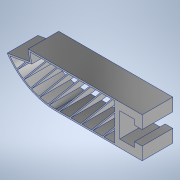
# Autodesk Inventor part: Finray_9_Kerbe_10deg_40deg10inf_PLA
Saved by Autodesk Inventor 2022 (Build 260153000, 153)
## iProperties
Created: 2022-02-28
Part Number: Finray_9_Kerbe_10deg_40deg10inf_PLA
Material: Generic
Document SubType Name: Modeling
Designer: richa
Density: 1 g/cm^3
Appearance: Aluminum - Flat
Author: richa
Autodesk Inventor part; units mm, degrees
ref_plane "YZ Plane" through (0, 0, 0) normal (1, 0, 0) x (0, 1, 0)
ref_plane "XZ Plane" through (0, 0, 0) normal (0, 1, 0) x (-1, 0, 0)
ref_plane "XY Plane" through (0, 0, 0) normal (0, 0, 1) x (1, 0, 0)
sketch "Sketch5" plane through (0, 0, 0) normal (0, 0, 1) x (1, 0, 0)
  line L0 (52.8, -15.6) -> (52.8, -10.6)
  line L1 (52.8, -10.6) -> (49.8, -10.6)
  line L2 (49.8, -10.6) -> (49.8, -12.6)
  line L3 (44, -12.6) -> (44, -3)
  line L4 (49.8, -3) -> (49.8, -5)
  line L5 (49.8, -5) -> (52.8, -5)
  line L6 (52.8, -5) -> (52.8, 0)
  line L7 (52.8, 0) -> (7.8, 0)
  line L8 (44, -3) -> (49.8, -3)
  line L9 (44, -12.6) -> (49.8, -12.6)
  line L10 (52.8, -15.6) -> (7.8, -15.6)
  line L11 (7.8, -15.6) -> (0, -15.6)
  line L12 (0, -15.6) -> (0, 0)
  line L13 (0, 0) -> (7.8, 0)
  point P0 (7.8, 0)
  dimension "d41" = 5.8
  dimension "d48" = 44
  dimension "d50" = 3
  dimension "d63" = 45
  dimension "d71" = 0
  dimension "d87" = 5.6
  dimension "d88" = 9.6
  dimension "d97" = 15.6
  constraints: 28 end point, 8 perpendicular, 4 collinear, 3 parallel, 2 horizontal, 1 vertical
  measures "d41" distance between parallel lines of L2 L3
  measures "d48" distance from line of L3 L12.end
  measures "d50" distance of L4.end L5.end
  measures "d63" distance of L0.start L10.end
  measures "d71" distance from line of L12.end L7
  measures "d87" distance from line of L0.end L5
  measures "d88" distance of L3.start L3.end
  measures "d97" distance of L11.end L12.end
extrude "Extrusion2" add sketch "Sketch5" along normal blind 12
sketch "Sketch8" plane through (0, 0, 0) normal (0, 0, -1) x (-1, 0, 0)
  line L0 (-8.1687, 0) -> (-8.8633, -3.9392)
  line L1 (-7.8, 0) -> (-1.143, 0) construction
  line L2 (0, -5.5021) -> (-8.8633, -3.9392)
  line L3 (-7.8, 0) -> (-8.1687, 0)
  line L4 (0, 0) -> (0, -15.6) projected
  line L5 (-52.8, 0) -> (0, 0) projected
  line L6 (-7.8, 0) -> (0, 0)
  line L7 (0, 0) -> (0, -5.5021)
  dimension "d80" = 100
  dimension "d95" = 4
  dimension "d96" = 9
  constraints: 12 end point, 2 collinear, 2 perpendicular, 1 horizontal, 1 point on line
  measures "d80" angle of L0 L1
  measures "d95" distance of L0.start L0.end
  measures "d96" distance of L2.start L0.end
extrude "Extrusion5" cut sketch "Sketch8" against normal through all
fillet "Fillet2" radius 23 1 edges at (0, -15.6, 6)
shell "Shell1" thickness 0.62 removed faces 1 at (23.9679, -7.5131, 12)
sketch "Sketch13" plane through (0, 0, 12) normal (0, 0, 1) x (1, 0, 0)
  line L0 (19.0404, -15.6) -> (52.8, -15.6) projected
  line L1 (42.0526, -15.6) -> (42.0526, 0)
  line L2 (52.8, 0) -> (8.1687, 0) projected
  line L3 (52.8, 0) -> (8.1687, 0) projected
  line L4 (52.8, -5) -> (52.8, 0) projected
  line L5 (49.8, -5) -> (52.8, -5) projected
  line L6 (49.8, -3) -> (49.8, -5) projected
  line L7 (44, -3) -> (49.8, -3) projected
  line L8 (44, -12.6) -> (44, -3) projected
  line L9 (49.8, -12.6) -> (44, -12.6) projected
  line L10 (49.8, -10.6) -> (49.8, -12.6) projected
  line L11 (52.8, -10.6) -> (49.8, -10.6) projected
  line L12 (52.8, -15.6) -> (52.8, -10.6) projected
  line L13 (42.0526, 0) -> (52.8, 0)
  line L14 (52.8, -5) -> (52.8, 0) projected
  line L15 (52.8, -5) -> (52.8, 0)
  line L16 (52.8, 0) -> (52.8, -5)
  line L17 (44, -12.6) -> (44, -3) projected
  line L18 (44, -3) -> (44, -12.6)
  line L19 (49.8, -12.6) -> (44, -12.6) projected
  line L20 (44, -12.6) -> (49.8, -12.6)
  line L21 (43.38, -13.22) -> (50.42, -13.22) projected
  line L22 (52.8, -10.6) -> (52.8, -15.6)
  line L23 (52.8, -15.6) -> (42.0526, -15.6)
  line L24 (44, -3) -> (49.8, -3) projected
  line L25 (44, -3) -> (49.8, -3)
  line L26 (49.8, -3) -> (49.8, -5)
  line L27 (49.8, -5) -> (52.8, -5)
  line L28 (52.8, -10.6) -> (49.8, -10.6)
  line L29 (49.8, -10.6) -> (49.8, -12.6)
  point P0 (0, 0)
  dimension "d102" = 10.7474
  constraints: 26 end point, 10 collinear, 2 point on line, 2 vertical, 1 parallel
  measures "d102" distance between parallel lines of L4 L1
extrude "Extrusion7" add sketch "Sketch13" against normal blind 12
sketch "Sketch14" plane through (8.9076, -0.62, 0.62) normal (0, 0, 1) x (1, 0, 0)
  line L0 (33.145, -14.36) -> (33.145, 0) projected
  line L1 (33.145, 0) -> (0, 0) projected
  line L2 (0.6739, -3.8221) -> (0, 0) projected
  line L3 (-7.835, -5.3225) -> (0.6739, -3.8221) projected
  arc A0 (-7.835, -5.3225) -> (10.1328, -14.36) centre (10.1328, 8.02) ccw projected
  line L4 (10.1328, -14.36) -> (33.145, -14.36) projected
  point P0 (-8.9076, 0.62)
extrude "Extrusion8" cut sketch "Sketch14" against normal blind 12
sketch "Sketch15" plane through (0, 0, 12) normal (0, 0, 1) x (1, 0, 0)
  line L0 (42.0526, -0.62) -> (8.9076, -0.62) construction
  line L1 (19.0404, -14.98) -> (42.0526, -14.98) projected
  line L2 (49.5848, -0.3757) -> (49.8759, -0.62)
  line L3 (49.8759, -0.62) -> (37.6215, -15.2243)
  line L4 (37.6215, -15.2243) -> (37.3304, -14.98)
  line L5 (37.3304, -14.98) -> (49.5848, -0.3757)
  arc A0 (1.0726, -5.9425) -> (19.0404, -14.98) centre (19.0404, 7.4) ccw projected
  line L6 (42.0526, -0.62) -> (42.0526, -14.98) projected
  line L7 (1.0726, -5.9425) -> (9.5815, -4.4421) projected
  arc A1 (0, -5.5021) -> (19.0404, -15.6) centre (19.0404, 7.4) ccw projected
  line L8 (42.0526, -14.98) -> (19.0404, -14.98) projected
  line L9 (8.9076, -0.62) -> (42.0526, -0.62) projected
  line L10 (45.5759, -0.62) -> (33.5265, -14.98)
  line L11 (45.0799, -0.62) -> (33.0304, -14.98)
  line L12 (36.9759, -0.62) -> (24.9265, -14.98)
  line L13 (36.4799, -0.62) -> (24.4304, -14.98)
  line L14 (32.6759, -0.62) -> (20.6265, -14.98)
  line L15 (32.1799, -0.62) -> (20.1304, -14.98)
  line L16 (28.3759, -0.62) -> (16.3265, -14.98)
  line L17 (27.8799, -0.62) -> (15.8304, -14.98)
  line L18 (24.0759, -0.62) -> (12.7769, -14.0856)
  line L19 (19.7759, -0.62) -> (9.5131, -12.8508)
  line L20 (19.2799, -0.62) -> (9.1597, -12.6807)
  line L21 (15.4759, -0.62) -> (6.5968, -11.2017)
  line L22 (14.9799, -0.62) -> (6.2812, -10.9866)
  line L23 (11.1759, -0.62) -> (3.9997, -9.1723)
  line L24 (10.6799, -0.62) -> (3.7202, -8.9143)
  line L25 (23.5799, -0.62) -> (12.381, -13.9663)
  line L26 (41.2759, -0.62) -> (29.2265, -14.98)
  line L27 (40.7799, -0.62) -> (28.7304, -14.98)
  point P0 (0, 0)
  point P1 (37.3304, -14.98)
  point P2 (7.6887, -4.7759)
  point P3 (7.1065, -4.8786)
  point P4 (37.8265, -14.98)
  point P5 (37.3304, -14.98)
  point P6 (33.0304, -14.98)
  point P7 (33.5265, -14.98)
  point P8 (28.7304, -14.98)
  point P9 (29.2265, -14.98)
  point P10 (24.4304, -14.98)
  point P11 (20.1304, -14.98)
  point P12 (20.6265, -14.98)
  point P13 (19.1926, -14.98)
  point P14 (19.4987, -14.98)
  point P15 (42.0526, -4.8189)
  point P16 (42.0526, -4.2278)
  point P17 (16.004, -14.7731)
  point P18 (16.4524, -14.8299)
  dimension "d105" = 0.38
  dimension "d130" = 130
  dimension "d132" = 130
  dimension "d133" = 0.38
  dimension "d135" = 0.38
  dimension "d136" = 0.38
  dimension "d137" = 0.38
  dimension "d138" = 0.38
  dimension "d139" = 0.38
  dimension "d140" = 0.38
  dimension "d141" = 0.38
  dimension "d143" = 0.38
  dimension "d152" = 130
  dimension "d155" = 4.3
  dimension "d156" = 4.3
  dimension "d157" = 4.3
  dimension "d158" = 4.3
  dimension "d159" = 4.3
  dimension "d160" = 4.3
  dimension "d161" = 4.3
  dimension "d162" = 4.3
  dimension "d164" = 4.3
  constraints: 44 end point, 18 parallel, 4 point on line, 1 perpendicular, 41 other
  measures "d105" distance between parallel lines of L3 L5
  measures "d130" angle of L0 L3
  measures "d132" angle of L0 L10
  measures "d133" distance between parallel lines of L10 L11
  measures "d135" distance between parallel lines of L13 L12
  measures "d136" distance between parallel lines of L15 L14
  measures "d137" distance between parallel lines of L17 L16
  measures "d138" distance between parallel lines of L25 L18
  measures "d139" distance between parallel lines of L20 L19
  measures "d140" distance between parallel lines of L22 L21
  measures "d141" distance between parallel lines of L24 L23
  measures "d143" distance between parallel lines of L26 L27
  measures "d152" angle of L0 L12
  measures "d155" distance of L10.start L2.end
  measures "d156" distance of L26.start L10.start
  measures "d157" distance of L12.start L26.start
  measures "d158" distance of L14.start L12.start
  measures "d159" distance of L16.start L14.start
  measures "d160" distance of L18.start L16.start
  measures "d161" distance of L19.start L18.start
  measures "d162" distance of L21.start L19.start
  measures "d164" distance of L23.start L21.start
extrude "Extrusion9" add sketch "Sketch15" against normal blind 12 contours L15 L9 L14 L1 | A0 L17 L9 L16 | L13 L9 L12 L1 | A0 L25 L9 L18 | L27 L9 L26 L1 | A0 L20 L9 L19 | L11 L6 L10 L1 | A0 L22 L9 L21 | L5 L6 L3 L1 | A0 L24 L7 L23 | L5 L2 L3 L6
sketch "Sketch16" plane through (0, 0, 12) normal (0, 0, 1) x (1, 0, 0)
  line L0 (49.8, -3) -> (49.8, -5) projected
  line L1 (44, -12.6) -> (49.8, -12.6)
  line L2 (49.8, -12.6) -> (49.8, -3)
  line L3 (49.8, -3) -> (44, -3)
  line L4 (44, -3) -> (44, -12.6)
  point P0 (0, 0)
  constraints: 8 end point, 2 parallel, 1 horizontal, 1 perpendicular
extrude "Extrusion10" cut sketch "Sketch16" against normal blind 12
equation "\"l1\" = 8"
equation "\"d1\" = 0.38"
body "Solid2"
